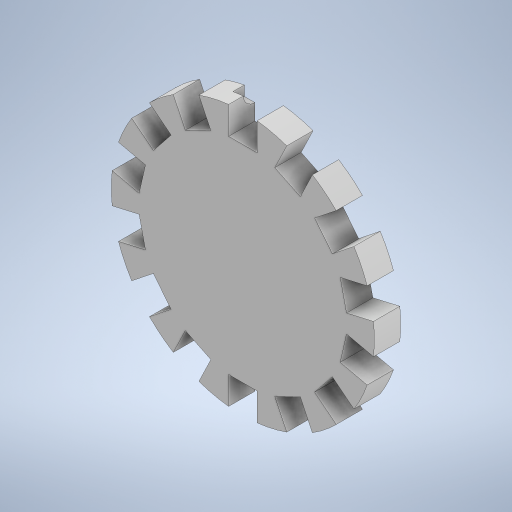
# Autodesk Inventor part: frame
Saved by Autodesk Inventor 2024.1 (Build 281209000, 209)
## iProperties
Created: 2024-06-29
Part Number: frame
Material: 一般
Document SubType Name: Modeling
Designer: hibik
Density: 1 g/cm^3
Appearance: 既定
Author: hibik
Autodesk Inventor part; units mm, degrees
ref_plane "YZ Plane" through (0, 0, 0) normal (1, 0, 0) x (0, 1, 0)
ref_plane "XZ Plane" through (0, 0, 0) normal (0, 1, 0) x (-1, 0, 0)
ref_plane "XY Plane" through (0, 0, 0) normal (0, 0, 1) x (1, 0, 0)
sketch "スケッチ1" plane through (0, 0, 0) normal (0, 0, 1) x (1, 0, 0)
  circle A0 centre (0, 0) radius 12.5
  line L0 (-1.35, 12.5) -> (1.35, 12.5) construction
  line L1 (1.35, 12.5) -> (1.35, 9.8)
  line L2 (1.35, 9.8) -> (-1.35, 9.8)
  line L3 (-1.35, 9.8) -> (-1.35, 12.5)
  line L4 (-5.4684, 8.2438) -> (-6.6399, 10.6764)
  line L5 (-4.2072, 11.8479) -> (-3.0358, 9.4152)
  line L6 (-3.0358, 9.4152) -> (-5.4684, 8.2438)
  line L7 (-8.5037, 5.0547) -> (-10.6146, 6.7382)
  line L8 (-8.9312, 8.8491) -> (-6.8202, 7.1657)
  line L9 (-6.8202, 7.1657) -> (-8.5037, 5.0547)
  line L10 (-9.8547, 0.8646) -> (-12.487, 1.4654)
  line L11 (-11.8862, 4.0977) -> (-9.2539, 3.4969)
  line L12 (-9.2539, 3.4969) -> (-9.8547, 0.8646)
  line L13 (-9.2539, -3.4969) -> (-11.8862, -4.0977)
  line L14 (-12.487, -1.4654) -> (-9.8547, -0.8646)
  line L15 (-9.8547, -0.8646) -> (-9.2539, -3.4969)
  line L16 (-6.8202, -7.1657) -> (-8.9312, -8.8491)
  line L17 (-10.6146, -6.7382) -> (-8.5037, -5.0547)
  line L18 (-8.5037, -5.0547) -> (-6.8202, -7.1657)
  line L19 (-3.0358, -9.4152) -> (-4.2072, -11.8479)
  line L20 (-6.6399, -10.6764) -> (-5.4684, -8.2438)
  line L21 (-5.4684, -8.2438) -> (-3.0358, -9.4152)
  line L22 (1.35, -9.8) -> (1.35, -12.5)
  line L23 (-1.35, -12.5) -> (-1.35, -9.8)
  line L24 (-1.35, -9.8) -> (1.35, -9.8)
  line L25 (5.4684, -8.2438) -> (6.6399, -10.6764)
  line L26 (4.2072, -11.8479) -> (3.0358, -9.4152)
  line L27 (3.0358, -9.4152) -> (5.4684, -8.2438)
  line L28 (8.5037, -5.0547) -> (10.6146, -6.7382)
  line L29 (8.9312, -8.8491) -> (6.8202, -7.1657)
  line L30 (6.8202, -7.1657) -> (8.5037, -5.0547)
  line L31 (9.8547, -0.8646) -> (12.487, -1.4654)
  line L32 (11.8862, -4.0977) -> (9.2539, -3.4969)
  line L33 (9.2539, -3.4969) -> (9.8547, -0.8646)
  line L34 (9.2539, 3.4969) -> (11.8862, 4.0977)
  line L35 (12.487, 1.4654) -> (9.8547, 0.8646)
  line L36 (9.8547, 0.8646) -> (9.2539, 3.4969)
  line L37 (6.8202, 7.1657) -> (8.9312, 8.8491)
  line L38 (10.6146, 6.7382) -> (8.5037, 5.0547)
  line L39 (8.5037, 5.0547) -> (6.8202, 7.1657)
  line L40 (3.0358, 9.4152) -> (4.2072, 11.8479)
  line L41 (6.6399, 10.6764) -> (5.4684, 8.2438)
  line L42 (5.4684, 8.2438) -> (3.0358, 9.4152)
  point P0 (0, 12.5)
  point P1 (-1.35, 12.4269)
  point P2 (-4.1755, 11.782)
  point P3 (-6.6081, 10.6105)
  point P4 (-8.874, 8.8035)
  point P5 (-10.5574, 6.6926)
  point P6 (-11.8149, 4.0814)
  point P7 (-12.4157, 1.4491)
  point P8 (-12.4157, -1.4491)
  point P9 (-11.8149, -4.0814)
  point P10 (-10.5574, -6.6926)
  point P11 (-8.874, -8.8035)
  point P12 (-6.6081, -10.6105)
  point P13 (-4.1755, -11.782)
  point P14 (-1.35, -12.4269)
  point P15 (1.35, -12.4269)
  point P16 (4.1755, -11.782)
  point P17 (6.6081, -10.6105)
  point P18 (8.874, -8.8035)
  point P19 (10.5574, -6.6926)
  point P20 (11.8149, -4.0814)
  point P21 (12.4157, -1.4491)
  point P22 (12.4157, 1.4491)
  point P23 (11.8149, 4.0814)
  point P24 (1.35, 12.4269)
  point P25 (10.5574, 6.6926)
  point P26 (8.874, 8.8035)
  point P27 (6.6081, 10.6105)
  point P28 (4.1755, 11.782)
  dimension "d0" = 25
  dimension "d3" = 2.7
  dimension "d4" = 2.7
  dimension "d7" = 360
  constraints: 86 end point, 2 horizontal, 2 parallel, 1 coincident, 1 midpoint, 1 perpendicular, 1 vertical alignment, 101 other
  measures "d3" distance of L1.end L2.end
  measures "d4" distance of L0.end L1.end
extrude "押し出し2" add sketch "スケッチ1" along normal blind 2.5 contours A0 L31 L33 L32 L28 L30 L29 L25 L27 L26 L22 L24 L23 L19 L21 L20 L16 L18 L17 L13 L15 L14 L10 L12 L11 L7 L9 L8 L4 L6 L5 L3 L2 L1 L40 L42 L41 L37 L39 L38 L34 L36 L35
sketch "スケッチ2" plane through (-1.35, 9.8, 0) normal (1, 0, 0) x (0, 0, -1)
  line L0 (0, 0) -> (0, 2.6269) projected
  circle A0 centre (0, 2.6269) radius 1.1
  point P0 (0, -9.8)
  dimension "d11" = 2.2
  constraints: 1 centre point
  measures "d11" diameter of A0
extrude "押し出し3" cut sketch "スケッチ2" against normal blind 1
